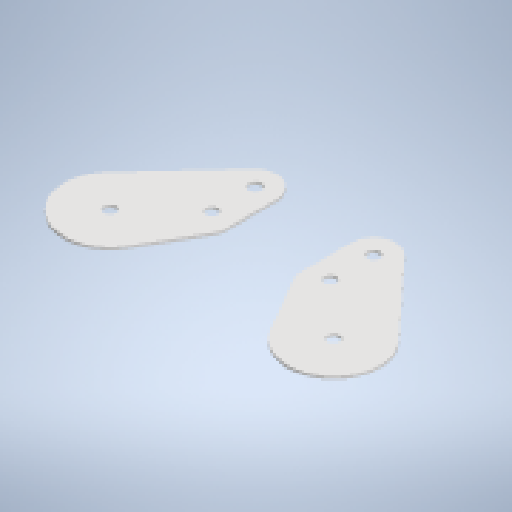
# Autodesk Inventor part: IntakeHolder
Saved by Autodesk Inventor 2023 (Build 270158000, 158)
## iProperties
Created: 2022-09-11
Part Number: IntakeHolder
Material: Generic
Document SubType Name: Modeling
Designer: deli
Density: 1 g/cm^3
Appearance: Default
Author: deli
Autodesk Inventor part; units mm, degrees
ref_plane "YZ Plane" through (0, 0, 0) normal (1, 0, 0) x (0, 1, 0)
ref_plane "XZ Plane" through (0, 0, 0) normal (0, 1, 0) x (-1, 0, 0)
ref_plane "XY Plane" through (0, 0, 0) normal (0, 0, 1) x (1, 0, 0)
sketch "Sketch1" plane through (0, 0, 0) normal (0, 1, 0) x (-1, 0, 0)
  circle A0 centre (21.4316, 162.4913) radius 7
  circle A1 centre (21.4316, 162.4913) radius 24 construction
  circle A2 centre (21.4316, 212.0913) radius 24 construction
  circle A3 centre (21.4316, 212.0913) radius 7
  circle A4 centre (157.4316, 162.4913) radius 7
  circle A5 centre (157.4316, 212.0913) radius 7
  circle A6 centre (157.4316, 212.0913) radius 24 construction
  circle A7 centre (157.4316, 162.4913) radius 24 construction
  line L0 (157.4316, 162.4913) -> (21.4316, 162.4913) construction
  line L1 (21.4316, 212.0913) -> (21.4316, 162.4913) construction
  line L2 (157.4316, 212.0913) -> (157.4316, 162.4913) construction
  circle A8 centre (89.4316, 131.3298) radius 50.8 construction
  arc A9 (3.1193, 145.4719) -> (46.4316, 162.4913) centre (21.4316, 162.4913) ccw
  arc A10 (132.4316, 162.4913) -> (175.7439, 145.4719) centre (157.4316, 162.4913) ccw
  line L3 (46.4316, 162.4913) -> (46.4316, 222.5028)
  line L4 (132.4316, 162.4913) -> (132.4316, 222.5028)
  circle A11 centre (-38.819, 268.4483) radius 48 construction
  line L5 (2.7502, 292.4483) -> (42.2162, 224.0913) construction
  circle A12 centre (-38.819, 268.4483) radius 7
  arc A13 (7.0803, 294.9483) -> (-77.6411, 232.3672) centre (-38.819, 268.4483) ccw
  line L6 (7.0803, 294.9483) -> (44.288, 230.5028)
  line L7 (-77.6411, 232.3672) -> (3.1193, 145.4719)
  circle A14 centre (217.6821, 268.4483) radius 7
  arc A15 (256.5042, 232.3672) -> (171.7828, 294.9483) centre (217.6821, 268.4483) ccw
  circle A16 centre (217.6821, 268.4483) radius 48 construction
  line L8 (176.1129, 292.4483) -> (136.647, 224.0913) construction
  line L9 (171.7828, 294.9483) -> (134.5752, 230.5028)
  line L10 (256.5042, 232.3672) -> (175.7439, 145.4719)
  circle A17 centre (89.4316, 193.6528) radius 50.8 construction
  arc A18 (134.5752, 230.5028) -> (132.4316, 222.5028) centre (148.4316, 222.5028) ccw
  arc A19 (46.4316, 222.5028) -> (44.288, 230.5028) centre (30.4316, 222.5028) ccw
  point P0 (0, 0)
  point P1 (46.4316, 226.79)
  point P2 (132.4316, 226.79)
  dimension "d2" = 48
  dimension "d5" = 48
  dimension "d26" = 96
  dimension "d32" = 96
  dimension "d36" = 88
  dimension "d0" = 14
  dimension "d1" = 48
  dimension "d3" = 14
  dimension "d4" = 49.6
  dimension "d6" = 14
  dimension "d7" = 14
  dimension "d8" = 48
  dimension "d9" = 49.6
  dimension "d10" = 88
  dimension "d11" = 90
  dimension "d12" = 90
  dimension "d13" = 101.6
  dimension "d21" = 86
  dimension "d27" = 82.5
  dimension "d28" = 120
  dimension "d29" = 14
  dimension "d30" = 5
  dimension "d31" = 14
  dimension "d33" = 5
  dimension "d34" = 120
  dimension "d35" = 82.5
  dimension "d37" = 101.6
  dimension "d38" = 16
  dimension "d39" = 16
  constraints: 22 end point, 16 centre point, 16 tangent, 12 point on circle, 10 coincident, 5 point on line, 2 parallel, 2 vertical, 1 equal radius, 1 horizontal, 16 other
  measures "d0" diameter of A0
  measures "d1" diameter of A1
  measures "d3" diameter of A3
  measures "d4" distance of A0.centre L1.start
  measures "d6" diameter of A5
  measures "d7" diameter of A4
  measures "d8" diameter of A7
  measures "d9" distance of A4.centre A5.centre
  measures "d11" angle of L0 L2
  measures "d12" angle of L0 L1
  measures "d13" diameter of A8
  measures "d21" distance between parallel lines of L4 L3
  measures "d27" distance of point (21.432, 212.091) point (-38.819, 268.448)
  measures "d28" angle of L0 L5
  measures "d29" diameter of A12
  measures "d31" diameter of A14
  measures "d34" angle of L0 L8
  measures "d35" distance of A5.centre A14.centre
  measures "d37" diameter of A17
  measures "d38" radius of A18
  measures "d39" radius of A19
extrude "Extrusion1" add sketch "Sketch1" along normal blind 3.175
equation "\"d2\" = d1"
equation "\"d5\" = d1"
equation "\"d32\" = d26"
equation "\"d3\" = d0"
equation "\"d6\" = d0"
equation "\"d7\" = d0"
equation "\"d8\" = d1"
equation "\"d9\" = d4"
equation "\"d12\" = d11"
equation "\"d30\" = d18"
equation "\"d31\" = d29"
equation "\"d33\" = d30"
equation "\"d34\" = d28"
equation "\"d35\" = d27"
equation "\"d37\" = d13"
equation "\"d39\" = d38"
equation "\"d17\" = d16"
equation "\"d18\" = 5"
equation "\"d16\" = 5"
body "Solid1"
